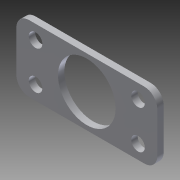
# Autodesk Inventor part: V5 Shooter Bearing Support Plate
Saved by Autodesk Inventor 2014 SP1 (Build 180222100, 222)
## iProperties
Created: 2012-02-08
Part Number: V5 Shooter Bearing Support Plate
Material: Aluminum-6061
Document SubType Name: Modeling
Designer: Moses
Mass: 12.7956 g
Surface Area: 41.4745 cm^2
Volume: 4.72162 cm^3
Density: 2.71 g/cm^3
Appearance: Aluminum - Flat
Author: Moses
Autodesk Inventor part; units mm, degrees
ref_plane "YZ Plane" through (0, 0, 0) normal (1, 0, 0) x (0, 1, 0)
ref_plane "XZ Plane" through (0, 0, 0) normal (0, 1, 0) x (-1, 0, 0)
ref_plane "XY Plane" through (0, 0, 0) normal (0, 0, 1) x (1, 0, 0)
sketch "Sketch1" plane through (0, 0, 0) normal (0, 0, 1) x (1, 0, 0)
  circle A0 centre (-194.945, 6.4301) radius 3.3782
  circle A1 centre (-194.945, 25.4801) radius 3.3782
  circle A2 centre (-144.145, 6.4301) radius 3.3782
  circle A3 centre (-144.145, 25.4801) radius 3.3782
  circle A4 centre (-169.545, 15.9551) radius 14.2875
  line L0 (-254, -1.8249) -> (254, -1.8249) construction
  line L1 (-247.65, 40.5304) -> (247.65, 40.5304) construction
  line L2 (-204.47, -0.5549) -> (-204.47, 32.4651)
  line L3 (-204.47, 32.4651) -> (-134.62, 32.4651)
  line L4 (-134.62, 32.4651) -> (-134.62, -0.5549)
  line L5 (-134.62, -0.5549) -> (-204.47, -0.5549)
  point P0 (0, 0)
extrude "Extrusion1" add sketch "Sketch1" along normal blind 3.175
fillet "Fillet1" radius 6.35 4 edges at (-204.47, 32.4651, 1.5875) (-204.47, -0.5549, 1.5875) (-134.62, 32.4651, 1.5875) (-134.62, -0.5549, 1.5875)
equation "\"d2\" = d1"
equation "\"d1\" = 9.525"
body "Solid1"
